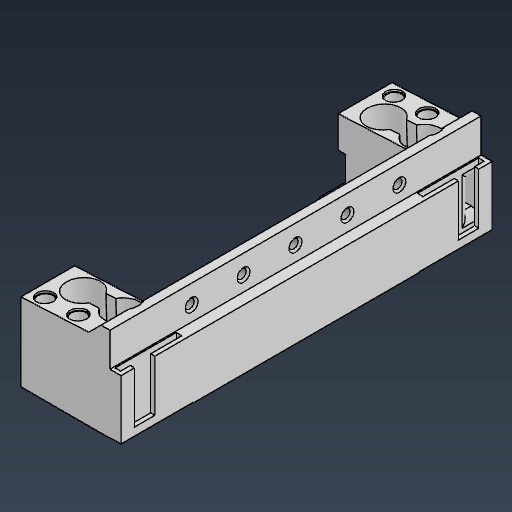
# Autodesk Inventor part: FonrtMount
Saved by Autodesk Inventor 2026.2 (Build 302298010, 298A)
## iProperties
Created: 2026-04-04
Part Number: FonrtMount
Material: Generic
Document SubType Name: Modeling
Designer: szymo
Density: 1 g/cm^3
Appearance: Default
Author: szymo
Autodesk Inventor part; units mm, degrees
(part 1 of 2)
ref_plane "YZ Plane" through (0, 0, 0) normal (1, 0, 0) x (0, 1, 0)
ref_plane "XZ Plane" through (0, 0, 0) normal (0, 1, 0) x (-1, 0, 0)
ref_plane "XY Plane" through (0, 0, 0) normal (0, 0, 1) x (1, 0, 0)
sketch "Sketch1" plane through (0, 0, 0) normal (0, 0, 1) x (1, 0, 0)
  line L0 (-27, 86.2958) -> (-6.5, 86.2958) projected
  line L1 (-6.5, 86.2958) -> (-6.5, 69.7958) projected
  line L2 (-27, 69.7958) -> (-6.5, 69.7958) projected
  line L3 (-27, 86.2958) -> (-27, 69.7958) projected
  line L4 (0, 95.9) -> (0, 81.9) projected
  line L5 (0, 81.9) -> (-3, 81.9) projected
  line L6 (-3, 81.9) -> (-3, 90.9) projected
  line L7 (-3, 90.9) -> (-5, 90.9) projected
  line L8 (-5, 90.9) -> (0, 95.9) projected
  circle A0 centre (-14.5, 55.2958) radius 14.5 projected
  line L9 (-9.2042, 86.6958) -> (-6, 86.6958)
  line L10 (-6, 86.6958) -> (-6, 69.2958)
  line L11 (-6, 69.2958) -> (-10.7251, 69.2958)
  line L12 (-4, 65.2958) -> (0, 65.2958)
  line L13 (0, 65.2958) -> (0, 81.4)
  line L14 (0, 81.4) -> (-3, 81.4)
  line L15 (-3, 81.4) -> (-3, 90.5)
  line L16 (-5.4, 90.5) -> (-9.2042, 86.6958)
  line L17 (-5.4, 90.5) -> (-3, 90.5)
  line L18 (-5.4, 90.5) -> (-5, 90.9) construction
  line L19 (-9.2085, 69.2958) -> (-9.2085, 68.7958)
  line L20 (-8.7042, 87.1958) -> (-8.7042, 86.6958)
  arc A1 (-5.2144, 40.6176) -> (-6.571, 40.1714) centre (-4.0302, 34.7325) ccw construction
  arc A2 (-4.9311, 40.2025) -> (-5.2144, 40.6176) centre (-13, 35.0012) ccw construction
  arc A3 (-5.8414, 39.102) -> (-4.9311, 40.2025) centre (-9.9791, 43.4512) ccw construction
  arc A4 (-5.6366, 38.7217) -> (-5.8414, 39.102) centre (-13, 35.0012) ccw construction
  arc A5 (-4.2168, 38.8762) -> (-5.6366, 38.7217) centre (-4.2821, 32.8735) ccw construction
  arc A6 (-4.026, 38.4112) -> (-4.2168, 38.8762) centre (-13, 35.0012) ccw construction
  arc A7 (-5.1452, 37.524) -> (-4.026, 38.4112) centre (-8.2882, 42.6385) ccw construction
  arc A8 (-5.0239, 37.1095) -> (-5.1452, 37.524) centre (-13, 35.0012) ccw construction
  arc A9 (-3.6031, 36.9654) -> (-5.0239, 37.1095) centre (-4.915, 31.1074) ccw construction
  arc A10 (-3.5132, 36.4709) -> (-3.6031, 36.9654) centre (-13, 35.0012) ccw construction
  arc A11 (-4.7923, 35.8358) -> (-3.5132, 36.4709) centre (-6.8033, 41.492) ccw construction
  arc A12 (-4.7599, 35.4051) -> (-4.7923, 35.8358) centre (-13, 35.0012) ccw construction
  arc A13 (-3.4001, 34.9687) -> (-4.7599, 35.4051) centre (-5.9012, 29.5115) ccw construction
  arc A14 (-3.4149, 34.4663) -> (-3.4001, 34.9687) centre (-13, 35.0012) ccw construction
  arc A15 (-4.7982, 34.1111) -> (-3.4149, 34.4663) centre (-5.5892, 40.0618) ccw construction
  arc A16 (-4.856, 33.6831) -> (-4.7982, 34.1111) centre (-13, 35.0012) ccw construction
  arc A17 (-3.6166, 32.9735) -> (-4.856, 33.6831) centre (-7.1977, 28.1556) ccw construction
  arc A18 (-3.7356, 32.4852) -> (-3.6166, 32.9735) centre (-13, 35.0012) ccw construction
  arc A19 (-5.1625, 32.4253) -> (-3.7356, 32.4852) centre (-4.699, 38.4104) ccw construction
  arc A20 (-5.308, 32.0186) -> (-5.1625, 32.4253) centre (-13, 35.0012) ccw construction
  arc A21 (-4.2432, 31.0669) -> (-5.308, 32.0186) centre (-8.7478, 27.0988) ccw construction
  arc A22 (-4.4611, 30.614) -> (-4.2432, 31.0669) centre (-13, 35.0012) ccw construction
  arc A23 (-5.8693, 30.8521) -> (-4.4611, 30.614) centre (-4.1716, 36.61) ccw construction
  arc A24 (-6.0962, 30.4845) -> (-5.8693, 30.8521) centre (-13, 35.0012) ccw construction
  arc A25 (-5.2526, 29.3322) -> (-6.0962, 30.4845) centre (-10.4837, 26.3874) ccw construction
  arc A26 (-5.5599, 28.9345) -> (-5.2526, 29.3322) centre (-13, 35.0012) ccw construction
  arc A27 (-6.8878, 29.4602) -> (-5.5599, 28.9345) centre (-4.03, 34.7394) ccw construction
  arc A28 (-7.1861, 29.1479) -> (-6.8878, 29.4602) centre (-13, 35.0012) ccw construction
  arc A29 (-6.6005, 27.8453) -> (-7.1861, 29.1479) centre (-12.3296, 26.0525) ccw construction
  arc A30 (-6.9838, 27.5202) -> (-6.6005, 27.8453) centre (-13, 35.0012) ccw construction
  arc A31 (-8.1734, 28.3104) -> (-6.9838, 27.5202) centre (-4.2805, 32.8801) ccw construction
  arc A32 (-8.5302, 28.067) -> (-8.1734, 28.3104) centre (-13, 35.0012) ccw construction
  arc A33 (-8.2282, 26.6712) -> (-8.5302, 28.067) centre (-14.2048, 26.1086) ccw construction
  arc A34 (-8.6707, 26.4328) -> (-8.2282, 26.6712) centre (-13, 35.0012) ccw construction
  arc A35 (-9.6699, 27.4531) -> (-8.6707, 26.4328) centre (-4.912, 31.1136) ccw construction
  arc A36 (-10.0695, 27.2892) -> (-9.6699, 27.4531) centre (-13, 35.0012) ccw construction
  arc A37 (-10.0643, 25.8611) -> (-10.0695, 27.2892) centre (-16.0273, 26.5534) ccw construction
  arc A38 (-10.5467, 25.72) -> (-10.0643, 25.8611) centre (-13, 35.0012) ccw construction
  arc A39 (-11.312, 26.9257) -> (-10.5467, 25.72) centre (-5.897, 29.5169) ccw construction
  arc A40 (-11.737, 26.8485) -> (-11.312, 26.9257) centre (-13, 35.0012) ccw construction
  arc A41 (-12.0288, 25.4504) -> (-11.737, 26.8485) centre (-17.7176, 27.3675) ccw construction
  arc A42 (-12.53, 25.4127) -> (-12.0288, 25.4504) centre (-13, 35.0012) ccw construction
  arc A43 (-13.0279, 26.7512) -> (-12.53, 25.4127) centre (-7.1925, 28.16) ccw construction
  arc A44 (-13.4596, 26.764) -> (-13.0279, 26.7512) centre (-13, 35.0012) ccw construction
  arc A45 (-14.0358, 25.4572) -> (-13.4596, 26.764) centre (-19.2016, 28.5151) ccw construction
  arc A46 (-14.5338, 25.5245) -> (-14.0358, 25.4572) centre (-13, 35.0012) ccw construction
  arc A47 (-14.7426, 26.9373) -> (-14.5338, 25.5245) centre (-8.7418, 27.102) ccw construction
  arc A48 (-15.1622, 27.0396) -> (-14.7426, 26.9373) centre (-13, 35.0012) ccw construction
  arc A49 (-15.9974, 25.8811) -> (-15.1622, 27.0396) centre (-20.4146, 29.9462) ccw construction
  arc A50 (-16.4706, 26.0505) -> (-15.9974, 25.8811) centre (-13, 35.0012) ccw construction
  arc A51 (-16.3811, 27.4758) -> (-16.4706, 26.0505) centre (-10.4772, 26.3893) ccw construction
  arc A52 (-16.7703, 27.6631) -> (-16.3811, 27.4758) centre (-13, 35.0012) ccw construction
  arc A53 (-17.8281, 26.7036) -> (-16.7703, 27.6631) centre (-21.3036, 31.5983) ccw construction
  arc A54 (-18.2557, 26.9677) -> (-17.8281, 26.7036) centre (-13, 35.0012) ccw construction
  arc A55 (-17.8718, 28.3432) -> (-18.2557, 26.9677) centre (-12.3228, 26.053) ccw construction
  arc A56 (-18.2136, 28.6073) -> (-17.8718, 28.3432) centre (-13, 35.0012) ccw construction
  arc A57 (-19.4477, 27.8888) -> (-18.2136, 28.6073) centre (-21.8296, 33.3991) ccw construction
  arc A58 (-19.8111, 28.236) -> (-19.4477, 27.8888) centre (-13, 35.0012) ccw construction
  arc A59 (-19.1496, 29.5016) -> (-19.8111, 28.236) centre (-14.198, 26.1077) ccw construction
  arc A60 (-19.429, 29.831) -> (-19.1496, 29.5016) centre (-13, 35.0012) ccw construction
  arc A61 (-20.7856, 29.3848) -> (-19.429, 29.831) centre (-21.9698, 35.2699) ccw construction
  arc A62 (-21.0689, 29.7999) -> (-20.7856, 29.3848) centre (-13, 35.0012) ccw construction
  arc A63 (-20.1586, 30.9004) -> (-21.0689, 29.7999) centre (-16.0209, 26.5512) ccw construction
  arc A64 (-20.3634, 31.2807) -> (-20.1586, 30.9004) centre (-13, 35.0012) ccw construction
  arc A65 (-21.7832, 31.1262) -> (-20.3634, 31.2807) centre (-21.7179, 37.1289) ccw construction
  arc A66 (-21.974, 31.5912) -> (-21.7832, 31.1262) centre (-13, 35.0012) ccw construction
  arc A67 (-20.8548, 32.4784) -> (-21.974, 31.5912) centre (-17.7118, 27.3639) ccw construction
  arc A68 (-20.9761, 32.8929) -> (-20.8548, 32.4784) centre (-13, 35.0012) ccw construction
  arc A69 (-22.3969, 33.037) -> (-20.9761, 32.8929) centre (-21.085, 38.895) ccw construction
  arc A70 (-22.4868, 33.5315) -> (-22.3969, 33.037) centre (-13, 35.0012) ccw construction
  arc A71 (-21.2077, 34.1666) -> (-22.4868, 33.5315) centre (-19.1967, 28.5104) ccw construction
  arc A72 (-21.2401, 34.5973) -> (-21.2077, 34.1666) centre (-13, 35.0012) ccw construction
  arc A73 (-22.5999, 35.0337) -> (-21.2401, 34.5973) centre (-20.0988, 40.4909) ccw construction
  arc A74 (-22.5851, 35.5361) -> (-22.5999, 35.0337) centre (-13, 35.0012) ccw construction
  arc A75 (-21.2018, 35.8913) -> (-22.5851, 35.5361) centre (-20.4108, 29.9406) ccw construction
  arc A76 (-21.144, 36.3193) -> (-21.2018, 35.8913) centre (-13, 35.0012) ccw construction
  arc A77 (-22.3834, 37.0289) -> (-21.144, 36.3193) centre (-18.8023, 41.8468) ccw construction
  arc A78 (-22.2644, 37.5172) -> (-22.3834, 37.0289) centre (-13, 35.0012) ccw construction
  arc A79 (-20.8375, 37.5771) -> (-22.2644, 37.5172) centre (-21.301, 31.592) ccw construction
  arc A80 (-20.692, 37.9838) -> (-20.8375, 37.5771) centre (-13, 35.0012) ccw construction
  arc A81 (-21.7568, 38.9355) -> (-20.692, 37.9838) centre (-17.2522, 42.9036) ccw construction
  arc A82 (-21.5389, 39.3884) -> (-21.7568, 38.9355) centre (-13, 35.0012) ccw construction
  arc A83 (-20.1307, 39.1503) -> (-21.5389, 39.3884) centre (-21.8284, 33.3924) ccw construction
  arc A84 (-19.9038, 39.5178) -> (-20.1307, 39.1503) centre (-13, 35.0012) ccw construction
  arc A85 (-20.7474, 40.6702) -> (-19.9038, 39.5178) centre (-15.5163, 43.615) ccw construction
  arc A86 (-20.4401, 41.0679) -> (-20.7474, 40.6702) centre (-13, 35.0012) ccw construction
  arc A87 (-19.1122, 40.5422) -> (-20.4401, 41.0679) centre (-21.97, 35.263) ccw construction
  arc A88 (-18.8139, 40.8545) -> (-19.1122, 40.5422) centre (-13, 35.0012) ccw construction
  arc A89 (-19.3995, 42.1571) -> (-18.8139, 40.8545) centre (-13.6704, 43.9499) ccw construction
  arc A90 (-19.0162, 42.4822) -> (-19.3995, 42.1571) centre (-13, 35.0012) ccw construction
  arc A91 (-17.8266, 41.692) -> (-19.0162, 42.4822) centre (-21.7195, 37.1223) ccw construction
  arc A92 (-17.4698, 41.9354) -> (-17.8266, 41.692) centre (-13, 35.0012) ccw construction
  arc A93 (-17.7718, 43.3312) -> (-17.4698, 41.9354) centre (-11.7952, 43.8938) ccw construction
  arc A94 (-17.3293, 43.5696) -> (-17.7718, 43.3312) centre (-13, 35.0012) ccw construction
  arc A95 (-16.3301, 42.5493) -> (-17.3293, 43.5696) centre (-21.088, 38.8888) ccw construction
  arc A96 (-15.9305, 42.7132) -> (-16.3301, 42.5493) centre (-13, 35.0012) ccw construction
  arc A97 (-15.9357, 44.1413) -> (-15.9305, 42.7132) centre (-9.9727, 43.4489) ccw construction
  arc A98 (-15.4533, 44.2824) -> (-15.9357, 44.1413) centre (-13, 35.0012) ccw construction
  arc A99 (-14.688, 43.0767) -> (-15.4533, 44.2824) centre (-20.103, 40.4855) ccw construction
  arc A100 (-14.263, 43.1539) -> (-14.688, 43.0767) centre (-13, 35.0012) ccw construction
  arc A101 (-13.9712, 44.5519) -> (-14.263, 43.1539) centre (-8.2824, 42.6349) ccw construction
  arc A102 (-13.47, 44.5897) -> (-13.9712, 44.5519) centre (-13, 35.0012) ccw construction
  arc A103 (-12.9721, 43.2512) -> (-13.47, 44.5897) centre (-18.8075, 41.8424) ccw construction
  arc A104 (-12.5404, 43.2384) -> (-12.9721, 43.2512) centre (-13, 35.0012) ccw construction
  arc A105 (-11.9642, 44.5452) -> (-12.5404, 43.2384) centre (-6.7984, 41.4873) ccw construction
  arc A106 (-11.4662, 44.4779) -> (-11.9642, 44.5452) centre (-13, 35.0012) ccw construction
  arc A107 (-11.2574, 43.0651) -> (-11.4662, 44.4779) centre (-17.2582, 42.9004) ccw construction
  arc A108 (-10.8378, 42.9628) -> (-11.2574, 43.0651) centre (-13, 35.0012) ccw construction
  arc A109 (-10.0026, 44.1213) -> (-10.8378, 42.9628) centre (-5.5854, 40.0562) ccw construction
  arc A110 (-9.5294, 43.9519) -> (-10.0026, 44.1213) centre (-13, 35.0012) ccw construction
  arc A111 (-9.6189, 42.5266) -> (-9.5294, 43.9519) centre (-15.5228, 43.6131) ccw construction
  arc A112 (-9.2297, 42.3393) -> (-9.6189, 42.5266) centre (-13, 35.0012) ccw construction
  arc A113 (-8.1719, 43.2988) -> (-9.2297, 42.3393) centre (-4.6964, 38.4041) ccw construction
  arc A114 (-7.7443, 43.0347) -> (-8.1719, 43.2988) centre (-13, 35.0012) ccw construction
  arc A115 (-8.1282, 41.6591) -> (-7.7443, 43.0347) centre (-13.6772, 43.9494) ccw construction
  arc A116 (-7.7864, 41.3951) -> (-8.1282, 41.6591) centre (-13, 35.0012) ccw construction
  arc A117 (-6.5523, 42.1136) -> (-7.7864, 41.3951) centre (-4.1704, 36.6033) ccw construction
  arc A118 (-6.1889, 41.7664) -> (-6.5523, 42.1136) centre (-13, 35.0012) ccw construction
  arc A119 (-6.8504, 40.5008) -> (-6.1889, 41.7664) centre (-11.802, 43.8947) ccw construction
  arc A120 (-6.571, 40.1714) -> (-6.8504, 40.5008) centre (-13, 35.0012) ccw construction
  circle A121 centre (-13, 35.0012) radius 9.6 construction
  line L21 (-4, 65.2958) -> (-27, 65.2958)
  line L22 (-27, 65.2958) -> (-27, 24.2538) construction
  line L23 (-27, 65.2958) -> (-27, 69.2958)
  line L24 (-27, 69.2958) -> (-9.2085, 69.2958)
  point P0 (0, 0)
  dimension "d0" = 4.5
  dimension "d1" = 0.5
  dimension "d2" = 0.5
  dimension "d3" = 0.4
  dimension "d4" = 45
  dimension "d5" = 0.4
  dimension "d6" = 0.5
  dimension "d11" = 0.5
  dimension "d12" = 0.5
  dimension "d32" = 2
  constraints: 32 end point, 7 perpendicular, 4 point on line, 3 horizontal, 3 point on circle, 3 vertical, 2 collinear, 1 coincident, 1 tangent, 3 other
  measures "d0" distance between parallel lines of L12 L2
  measures "d1" distance between parallel lines of L2 L11
  measures "d2" distance between parallel lines of L1 L10
  measures "d3" distance between parallel lines of L9 L0
  measures "d4" angle of L9 L16
  measures "d5" distance between parallel lines of L7 L17
  measures "d6" distance between parallel lines of L5 L14
  measures "d11" distance of L19.start L19.end
  measures "d12" distance of L20.start L20.end
  measures "d32" distance edge to line of A0 L22
extrude "Extrusion2" add sketch "Sketch1" along normal blind 19 and the other way blind 18.4 contours L19 L11 L10 L9 L20 L16 L17 L6 L15 L14 L13 L12 A0
sketch "Sketch2" plane through (0, 0, -18.4) normal (0, 0, -1) x (-1, 0, 0)
  arc A0 (6.571, 40.1714) -> (5.2144, 40.6176) centre (4.0302, 34.7325) ccw construction
  arc A1 (5.2144, 40.6176) -> (4.9311, 40.2025) centre (13, 35.0012) ccw construction
  arc A2 (4.9311, 40.2025) -> (5.8414, 39.102) centre (9.9791, 43.4512) ccw construction
  arc A3 (5.8414, 39.102) -> (5.6366, 38.7217) centre (13, 35.0012) ccw construction
  arc A4 (5.6366, 38.7217) -> (4.2168, 38.8762) centre (4.2821, 32.8735) ccw construction
  arc A5 (4.2168, 38.8762) -> (4.026, 38.4112) centre (13, 35.0012) ccw construction
  arc A6 (4.026, 38.4112) -> (5.1452, 37.524) centre (8.2882, 42.6385) ccw construction
  arc A7 (5.1452, 37.524) -> (5.0239, 37.1095) centre (13, 35.0012) ccw construction
  arc A8 (5.0239, 37.1095) -> (3.6031, 36.9654) centre (4.915, 31.1074) ccw construction
  arc A9 (3.6031, 36.9654) -> (3.5132, 36.4709) centre (13, 35.0012) ccw construction
  arc A10 (3.5132, 36.4709) -> (4.7923, 35.8358) centre (6.8033, 41.492) ccw construction
  arc A11 (4.7923, 35.8358) -> (4.7599, 35.4051) centre (13, 35.0012) ccw construction
  arc A12 (4.7599, 35.4051) -> (3.4001, 34.9687) centre (5.9012, 29.5115) ccw construction
  arc A13 (3.4001, 34.9687) -> (3.4149, 34.4663) centre (13, 35.0012) ccw construction
  arc A14 (3.4149, 34.4663) -> (4.7982, 34.1111) centre (5.5892, 40.0618) ccw construction
  arc A15 (4.7982, 34.1111) -> (4.856, 33.6831) centre (13, 35.0012) ccw construction
  arc A16 (4.856, 33.6831) -> (3.6166, 32.9735) centre (7.1977, 28.1556) ccw construction
  arc A17 (3.6166, 32.9735) -> (3.7356, 32.4852) centre (13, 35.0012) ccw construction
  arc A18 (3.7356, 32.4852) -> (5.1625, 32.4253) centre (4.699, 38.4104) ccw construction
  arc A19 (5.1625, 32.4253) -> (5.308, 32.0186) centre (13, 35.0012) ccw construction
  arc A20 (5.308, 32.0186) -> (4.2432, 31.0669) centre (8.7478, 27.0988) ccw construction
  arc A21 (4.2432, 31.0669) -> (4.4611, 30.614) centre (13, 35.0012) ccw construction
  arc A22 (4.4611, 30.614) -> (5.8693, 30.8521) centre (4.1716, 36.61) ccw construction
  arc A23 (5.8693, 30.8521) -> (6.0962, 30.4845) centre (13, 35.0012) ccw construction
  arc A24 (6.0962, 30.4845) -> (5.2526, 29.3322) centre (10.4837, 26.3874) ccw construction
  arc A25 (5.2526, 29.3322) -> (5.5599, 28.9345) centre (13, 35.0012) ccw construction
  arc A26 (5.5599, 28.9345) -> (6.8878, 29.4602) centre (4.03, 34.7394) ccw construction
  arc A27 (6.8878, 29.4602) -> (7.1861, 29.1479) centre (13, 35.0012) ccw construction
  arc A28 (7.1861, 29.1479) -> (6.6005, 27.8453) centre (12.3296, 26.0525) ccw construction
  arc A29 (6.6005, 27.8453) -> (6.9838, 27.5202) centre (13, 35.0012) ccw construction
  arc A30 (6.9838, 27.5202) -> (8.1734, 28.3104) centre (4.2805, 32.8801) ccw construction
  arc A31 (8.1734, 28.3104) -> (8.5302, 28.067) centre (13, 35.0012) ccw construction
  arc A32 (8.5302, 28.067) -> (8.2282, 26.6712) centre (14.2048, 26.1086) ccw construction
  arc A33 (8.2282, 26.6712) -> (8.6707, 26.4328) centre (13, 35.0012) ccw construction
  arc A34 (8.6707, 26.4328) -> (9.6699, 27.4531) centre (4.912, 31.1136) ccw construction
  arc A35 (9.6699, 27.4531) -> (10.0695, 27.2892) centre (13, 35.0012) ccw construction
  arc A36 (10.0695, 27.2892) -> (10.0643, 25.8611) centre (16.0273, 26.5534) ccw construction
  arc A37 (10.0643, 25.8611) -> (10.5467, 25.72) centre (13, 35.0012) ccw construction
  arc A38 (10.5467, 25.72) -> (11.312, 26.9257) centre (5.897, 29.5169) ccw construction
  arc A39 (11.312, 26.9257) -> (11.737, 26.8485) centre (13, 35.0012) ccw construction
  arc A40 (11.737, 26.8485) -> (12.0288, 25.4504) centre (17.7176, 27.3675) ccw construction
  arc A41 (12.0288, 25.4504) -> (12.53, 25.4127) centre (13, 35.0012) ccw construction
  arc A42 (12.53, 25.4127) -> (13.0279, 26.7512) centre (7.1925, 28.16) ccw construction
  arc A43 (13.0279, 26.7512) -> (13.4596, 26.764) centre (13, 35.0012) ccw construction
  arc A44 (13.4596, 26.764) -> (14.0358, 25.4572) centre (19.2016, 28.5151) ccw construction
  arc A45 (14.0358, 25.4572) -> (14.5338, 25.5245) centre (13, 35.0012) ccw construction
  arc A46 (14.5338, 25.5245) -> (14.7426, 26.9373) centre (8.7418, 27.102) ccw construction
  arc A47 (14.7426, 26.9373) -> (15.1622, 27.0396) centre (13, 35.0012) ccw construction
  arc A48 (15.1622, 27.0396) -> (15.9974, 25.8811) centre (20.4146, 29.9462) ccw construction
  arc A49 (15.9974, 25.8811) -> (16.4706, 26.0505) centre (13, 35.0012) ccw construction
  arc A50 (16.4706, 26.0505) -> (16.3811, 27.4758) centre (10.4772, 26.3893) ccw construction
  arc A51 (16.3811, 27.4758) -> (16.7703, 27.6631) centre (13, 35.0012) ccw construction
  arc A52 (16.7703, 27.6631) -> (17.8281, 26.7036) centre (21.3036, 31.5983) ccw construction
  arc A53 (17.8281, 26.7036) -> (18.2557, 26.9677) centre (13, 35.0012) ccw construction
  arc A54 (18.2557, 26.9677) -> (17.8718, 28.3432) centre (12.3228, 26.053) ccw construction
  arc A55 (17.8718, 28.3432) -> (18.2136, 28.6073) centre (13, 35.0012) ccw construction
  arc A56 (18.2136, 28.6073) -> (19.4477, 27.8888) centre (21.8296, 33.3991) ccw construction
  arc A57 (19.4477, 27.8888) -> (19.8111, 28.236) centre (13, 35.0012) ccw construction
  arc A58 (19.8111, 28.236) -> (19.1496, 29.5016) centre (14.198, 26.1077) ccw construction
  arc A59 (19.1496, 29.5016) -> (19.429, 29.831) centre (13, 35.0012) ccw construction
  arc A60 (19.429, 29.831) -> (20.7856, 29.3848) centre (21.9698, 35.2699) ccw construction
  arc A61 (20.7856, 29.3848) -> (21.0689, 29.7999) centre (13, 35.0012) ccw construction
  arc A62 (21.0689, 29.7999) -> (20.1586, 30.9004) centre (16.0209, 26.5512) ccw construction
  arc A63 (20.1586, 30.9004) -> (20.3634, 31.2807) centre (13, 35.0012) ccw construction
  arc A64 (20.3634, 31.2807) -> (21.7832, 31.1262) centre (21.7179, 37.1289) ccw construction
  arc A65 (21.7832, 31.1262) -> (21.974, 31.5912) centre (13, 35.0012) ccw construction
  arc A66 (21.974, 31.5912) -> (20.8548, 32.4784) centre (17.7118, 27.3639) ccw construction
  arc A67 (20.8548, 32.4784) -> (20.9761, 32.8929) centre (13, 35.0012) ccw construction
  arc A68 (20.9761, 32.8929) -> (22.3969, 33.037) centre (21.085, 38.895) ccw construction
  arc A69 (22.3969, 33.037) -> (22.4868, 33.5315) centre (13, 35.0012) ccw construction
  arc A70 (22.4868, 33.5315) -> (21.2077, 34.1666) centre (19.1967, 28.5104) ccw construction
  arc A71 (21.2077, 34.1666) -> (21.2401, 34.5973) centre (13, 35.0012) ccw construction
  arc A72 (21.2401, 34.5973) -> (22.5999, 35.0337) centre (20.0988, 40.4909) ccw construction
  arc A73 (22.5999, 35.0337) -> (22.5851, 35.5361) centre (13, 35.0012) ccw construction
  arc A74 (22.5851, 35.5361) -> (21.2018, 35.8913) centre (20.4108, 29.9406) ccw construction
  arc A75 (21.2018, 35.8913) -> (21.144, 36.3193) centre (13, 35.0012) ccw construction
  arc A76 (21.144, 36.3193) -> (22.3834, 37.0289) centre (18.8023, 41.8468) ccw construction
  arc A77 (22.3834, 37.0289) -> (22.2644, 37.5172) centre (13, 35.0012) ccw construction
  arc A78 (22.2644, 37.5172) -> (20.8375, 37.5771) centre (21.301, 31.592) ccw construction
  arc A79 (20.8375, 37.5771) -> (20.692, 37.9838) centre (13, 35.0012) ccw construction
  arc A80 (20.692, 37.9838) -> (21.7568, 38.9355) centre (17.2522, 42.9036) ccw construction
  arc A81 (21.7568, 38.9355) -> (21.5389, 39.3884) centre (13, 35.0012) ccw construction
  arc A82 (21.5389, 39.3884) -> (20.1307, 39.1503) centre (21.8284, 33.3924) ccw construction
  arc A83 (20.1307, 39.1503) -> (19.9038, 39.5178) centre (13, 35.0012) ccw construction
  arc A84 (19.9038, 39.5178) -> (20.7474, 40.6702) centre (15.5163, 43.615) ccw construction
  arc A85 (20.7474, 40.6702) -> (20.4401, 41.0679) centre (13, 35.0012) ccw construction
  arc A86 (20.4401, 41.0679) -> (19.1122, 40.5422) centre (21.97, 35.263) ccw construction
  arc A87 (19.1122, 40.5422) -> (18.8139, 40.8545) centre (13, 35.0012) ccw construction
  arc A88 (18.8139, 40.8545) -> (19.3995, 42.1571) centre (13.6704, 43.9499) ccw construction
  arc A89 (19.3995, 42.1571) -> (19.0162, 42.4822) centre (13, 35.0012) ccw construction
  arc A90 (19.0162, 42.4822) -> (17.8266, 41.692) centre (21.7195, 37.1223) ccw construction
  arc A91 (17.8266, 41.692) -> (17.4698, 41.9354) centre (13, 35.0012) ccw construction
  arc A92 (17.4698, 41.9354) -> (17.7718, 43.3312) centre (11.7952, 43.8938) ccw construction
  arc A93 (17.7718, 43.3312) -> (17.3293, 43.5696) centre (13, 35.0012) ccw construction
  arc A94 (17.3293, 43.5696) -> (16.3301, 42.5493) centre (21.088, 38.8888) ccw construction
  arc A95 (16.3301, 42.5493) -> (15.9305, 42.7132) centre (13, 35.0012) ccw construction
  arc A96 (15.9305, 42.7132) -> (15.9357, 44.1413) centre (9.9727, 43.4489) ccw construction
  arc A97 (15.9357, 44.1413) -> (15.4533, 44.2824) centre (13, 35.0012) ccw construction
  arc A98 (15.4533, 44.2824) -> (14.688, 43.0767) centre (20.103, 40.4855) ccw construction
  arc A99 (14.688, 43.0767) -> (14.263, 43.1539) centre (13, 35.0012) ccw construction
  arc A100 (14.263, 43.1539) -> (13.9712, 44.5519) centre (8.2824, 42.6349) ccw construction
  arc A101 (13.9712, 44.5519) -> (13.47, 44.5897) centre (13, 35.0012) ccw construction
  arc A102 (13.47, 44.5897) -> (12.9721, 43.2512) centre (18.8075, 41.8424) ccw construction
  arc A103 (12.9721, 43.2512) -> (12.5404, 43.2384) centre (13, 35.0012) ccw construction
  arc A104 (12.5404, 43.2384) -> (11.9642, 44.5452) centre (6.7984, 41.4873) ccw construction
  arc A105 (11.9642, 44.5452) -> (11.4662, 44.4779) centre (13, 35.0012) ccw construction
  arc A106 (11.4662, 44.4779) -> (11.2574, 43.0651) centre (17.2582, 42.9004) ccw construction
  arc A107 (11.2574, 43.0651) -> (10.8378, 42.9628) centre (13, 35.0012) ccw construction
  arc A108 (10.8378, 42.9628) -> (10.0026, 44.1213) centre (5.5854, 40.0562) ccw construction
  arc A109 (10.0026, 44.1213) -> (9.5294, 43.9519) centre (13, 35.0012) ccw construction
  arc A110 (9.5294, 43.9519) -> (9.6189, 42.5266) centre (15.5228, 43.6131) ccw construction
  arc A111 (9.6189, 42.5266) -> (9.2297, 42.3393) centre (13, 35.0012) ccw construction
  arc A112 (9.2297, 42.3393) -> (8.1719, 43.2988) centre (4.6964, 38.4041) ccw construction
  arc A113 (8.1719, 43.2988) -> (7.7443, 43.0347) centre (13, 35.0012) ccw construction
  arc A114 (7.7443, 43.0347) -> (8.1282, 41.6591) centre (13.6772, 43.9494) ccw construction
  arc A115 (8.1282, 41.6591) -> (7.7864, 41.3951) centre (13, 35.0012) ccw construction
  arc A116 (7.7864, 41.3951) -> (6.5523, 42.1136) centre (4.1704, 36.6033) ccw construction
  arc A117 (6.5523, 42.1136) -> (6.1889, 41.7664) centre (13, 35.0012) ccw construction
  arc A118 (6.1889, 41.7664) -> (6.8504, 40.5008) centre (11.802, 43.8947) ccw construction
  arc A119 (6.8504, 40.5008) -> (6.571, 40.1714) centre (13, 35.0012) ccw construction
  circle A120 centre (13, 35.0012) radius 9.6 construction
  line L0 (23.8, 32.6031) -> (23.8, 65.2958) construction
  line L1 (9.2085, 69.2958) -> (6, 69.2958) projected
  line L2 (6, 69.2958) -> (6, 86.6958) projected
  line L3 (6, 86.6958) -> (8.7042, 86.6958) projected
  line L4 (8.7042, 86.6958) -> (8.7042, 87.1958) projected
  line L5 (8.7042, 87.1958) -> (5.4, 90.5) projected
  line L6 (5.4, 90.5) -> (3, 90.5) projected
  line L7 (3, 90.5) -> (3, 81.4) projected
  line L8 (3, 81.4) -> (0, 81.4) projected
  line L9 (0, 81.4) -> (0, 65.2958) projected
  line L10 (0, 65.2958) -> (4, 65.2958) projected
  arc A121 (9.2085, 68.7958) -> (4, 65.2958) centre (14.5, 55.2958) ccw projected
  line L11 (9.2085, 68.7958) -> (9.2085, 69.2958) projected
  line L12 (4, 65.2958) -> (23.8, 65.2958)
  line L13 (23.8, 65.2958) -> (23.8, 69.2958)
  line L14 (23.8, 69.2958) -> (9.2085, 69.2958)
  circle A122 centre (14.5, 55.2958) radius 14.5 projected
  point P0 (0, 0)
  dimension "d33" = 5.2
  dimension "d35" = 1.2
  constraints: 8 end point, 2 vertical, 1 coincident, 1 horizontal, 1 perpendicular, 3 other
  measures "d33" distance edge to line of A122 L0
extrude "Extrusion3" add sketch "Sketch2" along normal blind 17.1 contours L11 A121 L10 L9 L8 L7 L6 L5 L4 L3 L2 L1 | L14 A122 L11 | A122 L14 L13 L12 A121 | L14 L13 A122
sketch "Sketch3" plane through (0, 0, 19) normal (0, 0, 1) x (1, 0, 0)
  arc A0 (-20.6322, 38.1335) -> (-22.0597, 38.1763) centre (-21.5245, 32.1971) ccw construction
  arc A1 (-22.0597, 38.1763) -> (-22.2135, 37.6978) centre (-13, 35.0012) ccw construction
  arc A2 (-22.2135, 37.6978) -> (-21.0283, 36.901) centre (-18.2955, 42.246) ccw construction
  arc A3 (-21.0283, 36.901) -> (-21.1167, 36.4782) centre (-13, 35.0012) ccw construction
  arc A4 (-21.1167, 36.4782) -> (-22.5219, 36.2233) centre (-20.7552, 30.4861) ccw construction
  arc A5 (-22.5219, 36.2233) -> (-22.5728, 35.7233) centre (-13, 35.0012) ccw construction
  arc A6 (-22.5728, 35.7233) -> (-21.2478, 35.1903) centre (-19.6861, 40.9866) ccw construction
  arc A7 (-21.2478, 35.1903) -> (-21.2464, 34.7584) centre (-13, 35.0012) ccw construction
  arc A8 (-21.2464, 34.7584) -> (-22.5679, 34.2168) centre (-19.647, 28.9724) ccw construction
  arc A9 (-22.5679, 34.2168) -> (-22.5137, 33.7172) centre (-13, 35.0012) ccw construction
  arc A10 (-22.5137, 33.7172) -> (-21.1069, 33.4714) centre (-20.7844, 39.4657) ccw construction
  arc A11 (-21.1069, 33.4714) -> (-21.0157, 33.0492) centre (-13, 35.0012) ccw construction
  arc A12 (-21.0157, 33.0492) -> (-22.1957, 32.2447) centre (-18.2483, 27.7221) ccw construction
  arc A13 (-22.1957, 32.2447) -> (-22.0389, 31.7672) centre (-13, 35.0012) ccw construction
  arc A14 (-22.0389, 31.7672) -> (-20.6117, 31.8193) centre (-21.5425, 37.7497) ccw construction
  arc A15 (-20.6117, 31.8193) -> (-20.4347, 31.4253) centre (-13, 35.0012) ccw construction
  arc A16 (-20.4347, 31.4253) -> (-21.4217, 30.393) centre (-16.6202, 26.79) ccw construction
  arc A17 (-21.4217, 30.393) -> (-21.169, 29.9586) centre (-13, 35.0012) ccw construction
  arc A18 (-21.169, 29.9586) -> (-19.7838, 30.3062) centre (-21.9273, 35.9136) ccw construction
  arc A19 (-19.7838, 30.3062) -> (-19.5288, 29.9576) centre (-13, 35.0012) ccw construction
  arc A20 (-19.5288, 29.9576) -> (-20.2796, 28.7428) centre (-14.8338, 26.2168) ccw construction
  arc A21 (-20.2796, 28.7428) -> (-19.9421, 28.3704) centre (-13, 35.0012) ccw construction
  arc A22 (-19.9421, 28.3704) -> (-18.6594, 28.9984) centre (-21.9219, 34.0375) ccw construction
  arc A23 (-18.6594, 28.9984) -> (-18.3375, 28.7104) centre (-13, 35.0012) ccw construction
  arc A24 (-18.3375, 28.7104) -> (-18.8193, 27.366) centre (-12.9674, 26.0275) ccw construction
  arc A25 (-18.8193, 27.366) -> (-18.4117, 27.0719) centre (-13, 35.0012) ccw construction
  arc A26 (-18.4117, 27.0719) -> (-17.2877, 27.9529) centre (-21.5266, 32.2036) ccw construction
  arc A27 (-17.2877, 27.9529) -> (-16.9129, 27.7382) centre (-13, 35.0012) ccw construction
  arc A28 (-16.9129, 27.7382) -> (-17.1047, 26.323) centre (-11.1024, 26.2303) ccw construction
  arc A29 (-17.1047, 26.323) -> (-16.6449, 26.12) centre (-13, 35.0012) ccw construction
  arc A30 (-16.6449, 26.12) -> (-15.7286, 27.2155) centre (-20.7586, 30.492) ccw construction
  arc A31 (-15.7286, 27.2155) -> (-15.3174, 27.0834) centre (-13, 35.0012) ccw construction
  arc A32 (-15.3174, 27.0834) -> (-15.2107, 25.6592) centre (-9.3203, 26.8165) ccw construction
  arc A33 (-15.2107, 25.6592) -> (-14.7187, 25.5563) centre (-13, 35.0012) ccw construction
  arc A34 (-14.7187, 25.5563) -> (-14.0502, 26.8183) centre (-19.6515, 28.9774) ccw construction
  arc A35 (-14.0502, 26.8183) -> (-13.6205, 26.7746) centre (-13, 35.0012) ccw construction
  arc A36 (-13.6205, 26.7746) -> (-13.2201, 25.4037) centre (-7.699, 27.7605) ccw construction
  arc A37 (-13.2201, 25.4037) -> (-12.7175, 25.4054) centre (-13, 35.0012) ccw construction
  arc A38 (-12.7175, 25.4054) -> (-12.3259, 26.7788) centre (-18.2538, 27.7261) ccw construction
  arc A39 (-12.3259, 26.7788) -> (-11.8965, 26.8253) centre (-13, 35.0012) ccw construction
  arc A40 (-11.8965, 26.8253) -> (-11.2198, 25.5677) centre (-6.3094, 29.0208) ccw construction
  arc A41 (-11.2198, 25.5677) -> (-10.7286, 25.6738) centre (-13, 35.0012) ccw construction
  arc A42 (-10.7286, 25.6738) -> (-10.6311, 27.0986) centre (-16.6264, 26.7928) ccw construction
  arc A43 (-10.6311, 27.0986) -> (-10.2208, 27.2334) centre (-13, 35.0012) ccw construction
  arc A44 (-10.2208, 27.2334) -> (-9.2974, 26.144) centre (-5.2122, 30.5426) ccw construction
  arc A45 (-9.2974, 26.144) -> (-8.8389, 26.3499) centre (-13, 35.0012) ccw construction
  arc A46 (-8.8389, 26.3499) -> (-9.0399, 27.7638) centre (-14.8405, 26.2182) ccw construction
  arc A47 (-9.0399, 27.7638) -> (-8.6665, 27.981) centre (-13, 35.0012) ccw construction
  arc A48 (-8.6665, 27.981) -> (-7.5368, 27.1073) centre (-4.4554, 32.2592) ccw construction
  arc A49 (-7.5368, 27.1073) -> (-7.1311, 27.4041) centre (-13, 35.0012) ccw construction
  arc A50 (-7.1311, 27.4041) -> (-7.6217, 28.7453) centre (-12.9742, 26.0274) ccw construction
  arc A51 (-7.6217, 28.7453) -> (-7.3016, 29.0354) centre (-13, 35.0012) ccw construction
  arc A52 (-7.3016, 29.0354) -> (-6.0149, 28.4157) centre (-4.072, 34.0956) ccw construction
  arc A53 (-6.0149, 28.4157) -> (-5.6799, 28.7903) centre (-13, 35.0012) ccw construction
  arc A54 (-5.6799, 28.7903) -> (-6.4385, 30.0002) centre (-11.109, 26.2289) ccw construction
  arc A55 (-6.4385, 30.0002) -> (-6.1858, 30.3505) centre (-13, 35.0012) ccw construction
  arc A56 (-6.1858, 30.3505) -> (-4.7984, 30.0119) centre (-4.0788, 35.9716) ccw construction
  arc A57 (-4.7984, 30.0119) -> (-4.5485, 30.448) centre (-13, 35.0012) ccw construction
  arc A58 (-4.5485, 30.448) -> (-5.5422, 31.4737) centre (-9.3265, 26.8137) ccw construction
  arc A59 (-5.5422, 31.4737) -> (-5.3678, 31.8689) centre (-13, 35.0012) ccw construction
  arc A60 (-5.3678, 31.8689) -> (-3.9403, 31.8261) centre (-4.4755, 37.8053) ccw construction
  arc A61 (-3.9403, 31.8261) -> (-3.7865, 32.3046) centre (-13, 35.0012) ccw construction
  arc A62 (-3.7865, 32.3046) -> (-4.9717, 33.1014) centre (-7.7045, 27.7564) ccw construction
  arc A63 (-4.9717, 33.1014) -> (-4.8833, 33.5242) centre (-13, 35.0012) ccw construction
  arc A64 (-4.8833, 33.5242) -> (-3.4781, 33.7791) centre (-5.2448, 39.5163) ccw construction
  arc A65 (-3.4781, 33.7791) -> (-3.4272, 34.2791) centre (-13, 35.0012) ccw construction
  arc A66 (-3.4272, 34.2791) -> (-4.7522, 34.8121) centre (-6.3139, 29.0157) ccw construction
  arc A67 (-4.7522, 34.8121) -> (-4.7536, 35.244) centre (-13, 35.0012) ccw construction
  arc A68 (-4.7536, 35.244) -> (-3.4321, 35.7855) centre (-6.353, 41.03) ccw construction
  arc A69 (-3.4321, 35.7855) -> (-3.4863, 36.2852) centre (-13, 35.0012) ccw construction
  arc A70 (-3.4863, 36.2852) -> (-4.8931, 36.531) centre (-5.2156, 30.5367) ccw construction
  arc A71 (-4.8931, 36.531) -> (-4.9843, 36.9532) centre (-13, 35.0012) ccw construction
  arc A72 (-4.9843, 36.9532) -> (-3.8043, 37.7577) centre (-7.7517, 42.2803) ccw construction
  arc A73 (-3.8043, 37.7577) -> (-3.9611, 38.2352) centre (-13, 35.0012) ccw construction
  arc A74 (-3.9611, 38.2352) -> (-5.3883, 38.1831) centre (-4.4575, 32.2527) ccw construction
  arc A75 (-5.3883, 38.1831) -> (-5.5653, 38.5771) centre (-13, 35.0012) ccw construction
  arc A76 (-5.5653, 38.5771) -> (-4.5783, 39.6094) centre (-9.3798, 43.2124) ccw construction
  arc A77 (-4.5783, 39.6094) -> (-4.831, 40.0438) centre (-13, 35.0012) ccw construction
  arc A78 (-4.831, 40.0438) -> (-6.2162, 39.6962) centre (-4.0727, 34.0888) ccw construction
  arc A79 (-6.2162, 39.6962) -> (-6.4712, 40.0448) centre (-13, 35.0012) ccw construction
  arc A80 (-6.4712, 40.0448) -> (-5.7204, 41.2596) centre (-11.1662, 43.7856) ccw construction
  arc A81 (-5.7204, 41.2596) -> (-6.0579, 41.632) centre (-13, 35.0012) ccw construction
  arc A82 (-6.0579, 41.632) -> (-7.3406, 41.004) centre (-4.0781, 35.9649) ccw construction
  arc A83 (-7.3406, 41.004) -> (-7.6625, 41.292) centre (-13, 35.0012) ccw construction
  arc A84 (-7.6625, 41.292) -> (-7.1807, 42.6364) centre (-13.0326, 43.9749) ccw construction
  arc A85 (-7.1807, 42.6364) -> (-7.5883, 42.9305) centre (-13, 35.0012) ccw construction
  arc A86 (-7.5883, 42.9305) -> (-8.7123, 42.0495) centre (-4.4734, 37.7988) ccw construction
  arc A87 (-8.7123, 42.0495) -> (-9.0871, 42.2642) centre (-13, 35.0012) ccw construction
  arc A88 (-9.0871, 42.2642) -> (-8.8953, 43.6794) centre (-14.8976, 43.7721) ccw construction
  arc A89 (-8.8953, 43.6794) -> (-9.3551, 43.8824) centre (-13, 35.0012) ccw construction
  arc A90 (-9.3551, 43.8824) -> (-10.2714, 42.7869) centre (-5.2414, 39.5104) ccw construction
  arc A91 (-10.2714, 42.7869) -> (-10.6826, 42.919) centre (-13, 35.0012) ccw construction
  arc A92 (-10.6826, 42.919) -> (-10.7893, 44.3432) centre (-16.6797, 43.1859) ccw construction
  arc A93 (-10.7893, 44.3432) -> (-11.2813, 44.4461) centre (-13, 35.0012) ccw construction
  arc A94 (-11.2813, 44.4461) -> (-11.9498, 43.1841) centre (-6.3485, 41.025) ccw construction
  arc A95 (-11.9498, 43.1841) -> (-12.3795, 43.2278) centre (-13, 35.0012) ccw construction
  arc A96 (-12.3795, 43.2278) -> (-12.7799, 44.5987) centre (-18.301, 42.2419) ccw construction
  arc A97 (-12.7799, 44.5987) -> (-13.2825, 44.597) centre (-13, 35.0012) ccw construction
  arc A98 (-13.2825, 44.597) -> (-13.6741, 43.2236) centre (-7.7462, 42.2763) ccw construction
  arc A99 (-13.6741, 43.2236) -> (-14.1035, 43.1771) centre (-13, 35.0012) ccw construction
  arc A100 (-14.1035, 43.1771) -> (-14.7802, 44.4347) centre (-19.6906, 40.9816) ccw construction
  arc A101 (-14.7802, 44.4347) -> (-15.2714, 44.3286) centre (-13, 35.0012) ccw construction
  arc A102 (-15.2714, 44.3286) -> (-15.3689, 42.9038) centre (-9.3736, 43.2096) ccw construction
  arc A103 (-15.3689, 42.9038) -> (-15.7792, 42.769) centre (-13, 35.0012) ccw construction
  arc A104 (-15.7792, 42.769) -> (-16.7026, 43.8584) centre (-20.7878, 39.4598) ccw construction
  arc A105 (-16.7026, 43.8584) -> (-17.1611, 43.6525) centre (-13, 35.0012) ccw construction
  arc A106 (-17.1611, 43.6525) -> (-16.9601, 42.2386) centre (-11.1595, 43.7842) ccw construction
  arc A107 (-16.9601, 42.2386) -> (-17.3335, 42.0214) centre (-13, 35.0012) ccw construction
  arc A108 (-17.3335, 42.0214) -> (-18.4632, 42.8951) centre (-21.5446, 37.7432) ccw construction
  arc A109 (-18.4632, 42.8951) -> (-18.8689, 42.5983) centre (-13, 35.0012) ccw construction
  arc A110 (-18.8689, 42.5983) -> (-18.3783, 41.2571) centre (-13.0258, 43.975) ccw construction
  arc A111 (-18.3783, 41.2571) -> (-18.6984, 40.967) centre (-13, 35.0012) ccw construction
  arc A112 (-18.6984, 40.967) -> (-19.9851, 41.5867) centre (-21.928, 35.9068) ccw construction
  arc A113 (-19.9851, 41.5867) -> (-20.3201, 41.2121) centre (-13, 35.0012) ccw construction
  arc A114 (-20.3201, 41.2121) -> (-19.5615, 40.0022) centre (-14.891, 43.7735) ccw construction
  arc A115 (-19.5615, 40.0022) -> (-19.8142, 39.6519) centre (-13, 35.0012) ccw construction
  arc A116 (-19.8142, 39.6519) -> (-21.2016, 39.9905) centre (-21.9212, 34.0308) ccw construction
  arc A117 (-21.2016, 39.9905) -> (-21.4515, 39.5544) centre (-13, 35.0012) ccw construction
  arc A118 (-21.4515, 39.5544) -> (-20.4578, 38.5287) centre (-16.6735, 43.1886) ccw construction
  arc A119 (-20.4578, 38.5287) -> (-20.6322, 38.1335) centre (-13, 35.0012) ccw construction
  line L0 (-6, 69.2958) -> (-9.2085, 69.2958) projected
  line L1 (-9.2085, 69.2958) -> (-9.2085, 68.7958) projected
  arc A120 (-4, 65.2958) -> (-9.2085, 68.7958) centre (-14.5, 55.2958) ccw projected
  line L2 (-4, 65.2958) -> (0, 65.2958) projected
  line L3 (0, 65.2958) -> (0, 81.4) projected
  line L4 (0, 81.4) -> (-3, 81.4) projected
  line L5 (-3, 81.4) -> (-3, 90.5) projected
  line L6 (-3, 90.5) -> (-5.4, 90.5) projected
  line L7 (-5.4, 90.5) -> (-8.7042, 87.1958) projected
  line L8 (-8.7042, 87.1958) -> (-8.7042, 86.6958) projected
  line L9 (-8.7042, 86.6958) -> (-6, 86.6958) projected
  line L10 (-6, 86.6958) -> (-6, 69.2958) projected
  circle A121 centre (-13, 35.0012) radius 9.6
  line L11 (-23.8, 30.4052) -> (-23.8, 69.2958)
  line L12 (-23.8, 69.2958) -> (-9.2085, 69.2958)
  line L13 (-4, 65.2958) -> (-23.8, 65.2958) projected
  line L14 (-4, 65.2958) -> (-23.8, 65.2958)
  circle A122 centre (-14.5, 55.2958) radius 14.5 projected
  point P0 (0, 0)
  point P1 (-25.5572, 65.2958)
  dimension "d34" = 5.2
  dimension "d36" = 1.2
  constraints: 6 end point, 2 perpendicular, 1 coincident, 1 vertical, 3 other
  measures "d34" distance edge to line of A122 L11
extrude "Extrusion4" add sketch "Sketch3" along normal blind 16.5 contours L10 L9 L8 L7 L6 L5 L4 L3 L2 A120 L1 L0 | L1 A122 L12 | A120 L13 L11 A122 L12 | A122 L11 L12
sketch "Sketch4" plane through (0, 0, -35.5) normal (0, 0, -1) x (-1, 0, 0)
  line L0 (26.0532, 64.5637) -> (22.0556, 64.7033)
  line L1 (5.4157, 65.2843) -> (22.0556, 64.7033)
  line L2 (5.4157, 65.2843) -> (1.4182, 65.4239)
  line L3 (23.8, 65.2958) -> (23.8, 69.2958)
  line L4 (23.8, 69.2958) -> (6, 69.2958)
  line L5 (6, 69.2958) -> (6, 86.6958)
  line L6 (6, 86.6958) -> (8.7042, 86.6958)
  line L7 (8.7042, 86.6958) -> (8.7042, 87.1958)
  line L8 (8.7042, 87.1958) -> (5.4, 90.5)
  line L9 (5.4, 90.5) -> (3, 90.5)
  line L10 (3, 90.5) -> (3, 81.4)
  line L11 (3, 81.4) -> (0, 81.4)
  line L12 (0, 81.4) -> (0, 65.2958)
  line L13 (0, 65.2958) -> (23.8, 65.2958)
  line L14 (1.4182, 65.4239) -> (0, 65.4735)
  line L15 (27, 52.5631) -> (27, 86.2958)
  line L16 (27, 86.2958) -> (8.7042, 87.1958)
  line L17 (27, 86.2958) -> (6.5, 86.2958)
  line L18 (26.0532, 64.5637) -> (27, 64.5306)
  line L19 (23.8, 65.2958) -> (23.8, 69.2958)
  arc A0 (18.7931, 40.8751) -> (19.3741, 42.1797) centre (13.6387, 43.9522) ccw
  arc A1 (19.3741, 42.1797) -> (18.9897, 42.5035) centre (13, 35.0012) ccw
  arc A2 (18.9897, 42.5035) -> (17.8029, 41.709) centre (21.712, 37.1532) ccw
  arc A3 (17.8029, 41.709) -> (17.4452, 41.9512) centre (13, 35.0012) ccw
  arc A4 (17.4452, 41.9512) -> (17.7423, 43.3481) centre (11.7637, 43.8894) ccw
  arc A5 (17.7423, 43.3481) -> (17.299, 43.5848) centre (13, 35.0012) ccw
  arc A6 (17.299, 43.5848) -> (16.3033, 42.561) centre (21.0742, 38.9175) ccw
  arc A7 (16.3033, 42.561) -> (15.9031, 42.7235) centre (13, 35.0012) ccw
  arc A8 (15.9031, 42.7235) -> (15.9033, 44.1517) centre (9.9428, 43.4382) ccw
  arc A9 (15.9033, 44.1517) -> (15.4204, 44.2911) centre (13, 35.0012) ccw
  arc A10 (15.4204, 44.2911) -> (14.6593, 43.0826) centre (20.0835, 40.5106) ccw
  arc A11 (14.6593, 43.0826) -> (14.2341, 43.1584) centre (13, 35.0012) ccw
  arc A12 (14.2341, 43.1584) -> (13.9373, 44.5553) centre (8.2554, 42.6182) ccw
  arc A13 (13.9373, 44.5553) -> (13.436, 44.5913) centre (13, 35.0012) ccw
  arc A14 (13.436, 44.5913) -> (12.9429, 43.251) centre (18.7832, 41.8629) ccw
  arc A15 (12.9429, 43.251) -> (12.5112, 43.2367) centre (13, 35.0012) ccw
  arc A16 (12.5112, 43.2367) -> (11.9304, 44.5414) centre (6.7755, 41.4653) ccw
  arc A17 (11.9304, 44.5414) -> (11.4326, 44.4724) centre (13, 35.0012) ccw
  arc A18 (11.4326, 44.4724) -> (11.2289, 43.0588) centre (17.2302, 42.9154) ccw
  arc A19 (11.2289, 43.0588) -> (10.8096, 42.9551) centre (13, 35.0012) ccw
  arc A20 (10.8096, 42.9551) -> (9.9703, 44.1106) centre (5.5675, 40.0299) ccw
  arc A21 (9.9703, 44.1106) -> (9.4977, 43.9395) centre (13, 35.0012) ccw
  arc A22 (9.4977, 43.9395) -> (9.5923, 42.5145) centre (15.4923, 43.622) ccw
  arc A23 (9.5923, 42.5145) -> (9.2038, 42.3259) centre (13, 35.0012) ccw
  arc A24 (9.2038, 42.3259) -> (8.1425, 43.2816) centre (4.6844, 38.3747) ccw
  arc A25 (8.1425, 43.2816) -> (7.7158, 43.016) centre (13, 35.0012) ccw
  arc A26 (7.7158, 43.016) -> (8.1047, 41.6418) centre (13.6455, 43.9518) ccw
  arc A27 (8.1047, 41.6418) -> (7.7638, 41.3765) centre (13, 35.0012) ccw
  arc A28 (7.7638, 41.3765) -> (6.5271, 42.0907) centre (4.1648, 36.572) ccw
  arc A29 (6.5271, 42.0907) -> (6.1649, 41.7423) centre (13, 35.0012) ccw
  arc A30 (6.1649, 41.7423) -> (6.831, 40.4789) centre (11.7705, 43.8904) ccw
  arc A31 (6.831, 40.4789) -> (6.5527, 40.1486) centre (13, 35.0012) ccw
  arc A32 (6.5527, 40.1486) -> (5.1945, 40.59) centre (4.0312, 34.7008) ccw
  arc A33 (5.1945, 40.59) -> (4.9127, 40.1739) centre (13, 35.0012) ccw
  arc A34 (4.9127, 40.1739) -> (5.8269, 39.0766) centre (9.9492, 43.4405) ccw
  arc A35 (5.8269, 39.0766) -> (5.6234, 38.6956) centre (13, 35.0012) ccw
  arc A36 (5.6234, 38.6956) -> (4.2031, 38.845) centre (4.2897, 32.8426) ccw
  arc A37 (4.2031, 38.845) -> (4.014, 38.3794) centre (13, 35.0012) ccw
  arc A38 (4.014, 38.3794) -> (5.1363, 37.4962) centre (8.2612, 42.6218) ccw
  arc A39 (5.1363, 37.4962) -> (5.0165, 37.0812) centre (13, 35.0012) ccw
  arc A40 (5.0165, 37.0812) -> (3.5962, 36.9321) centre (4.9288, 31.0788) ccw
  arc A41 (3.5962, 36.9321) -> (3.508, 36.4373) centre (13, 35.0012) ccw
  arc A42 (3.508, 36.4373) -> (4.7894, 35.8067) centre (6.7804, 41.47) ccw
  arc A43 (4.7894, 35.8067) -> (4.7585, 35.3759) centre (13, 35.0012) ccw
  arc A44 (4.7585, 35.3759) -> (3.4002, 34.9347) centre (5.9207, 29.4864) ccw
  arc A45 (3.4002, 34.9347) -> (3.4169, 34.4324) centre (13, 35.0012) ccw
  arc A46 (3.4169, 34.4324) -> (4.8014, 34.082) centre (5.5713, 40.0355) ccw
  arc A47 (4.8014, 34.082) -> (4.8607, 33.6542) centre (13, 35.0012) ccw
  arc A48 (4.8607, 33.6542) -> (3.6238, 32.9403) centre (7.222, 28.1351) ccw
  arc A49 (3.6238, 32.9403) -> (3.7445, 32.4524) centre (13, 35.0012) ccw
  arc A50 (3.7445, 32.4524) -> (5.1716, 32.3975) centre (4.687, 38.381) ccw
  arc A51 (5.1716, 32.3975) -> (5.3186, 31.9914) centre (13, 35.0012) ccw
  arc A52 (5.3186, 31.9914) -> (4.2572, 31.0359) centre (8.7758, 27.0838) ccw
  arc A53 (4.2572, 31.0359) -> (4.4767, 30.5838) centre (13, 35.0012) ccw
  arc A54 (4.4767, 30.5838) -> (5.884, 30.8268) centre (4.1659, 36.5788) ccw
  arc A55 (5.884, 30.8268) -> (6.1122, 30.4601) centre (13, 35.0012) ccw
  arc A56 (6.1122, 30.4601) -> (5.2727, 29.3048) centre (10.5142, 26.3786) ccw
  arc A57 (5.2727, 29.3048) -> (5.5814, 28.9082) centre (13, 35.0012) ccw
  arc A58 (5.5814, 28.9082) -> (6.9074, 29.4385) centre (4.031, 34.7076) ccw
  arc A59 (6.9074, 29.4385) -> (7.2069, 29.1273) centre (13, 35.0012) ccw
  arc A60 (7.2069, 29.1273) -> (6.6259, 27.8227) centre (12.3613, 26.0502) ccw
  arc A61 (6.6259, 27.8227) -> (7.0103, 27.4989) centre (13, 35.0012) ccw
  arc A62 (7.0103, 27.4989) -> (8.1971, 28.2934) centre (4.288, 32.8492) ccw
  arc A63 (8.1971, 28.2934) -> (8.5548, 28.0512) centre (13, 35.0012) ccw
  arc A64 (8.5548, 28.0512) -> (8.2577, 26.6543) centre (14.2363, 26.113) ccw
  arc A65 (8.2577, 26.6543) -> (8.701, 26.4176) centre (13, 35.0012) ccw
  arc A66 (8.701, 26.4176) -> (9.6967, 27.4414) centre (4.9258, 31.0849) ccw
  arc A67 (9.6967, 27.4414) -> (10.0969, 27.2789) centre (13, 35.0012) ccw
  arc A68 (10.0969, 27.2789) -> (10.0967, 25.8507) centre (16.0572, 26.5642) ccw
  arc A69 (10.0967, 25.8507) -> (10.5796, 25.7113) centre (13, 35.0012) ccw
  arc A70 (10.5796, 25.7113) -> (11.3407, 26.9198) centre (5.9165, 29.4918) ccw
  arc A71 (11.3407, 26.9198) -> (11.7659, 26.844) centre (13, 35.0012) ccw
  arc A72 (11.7659, 26.844) -> (12.0627, 25.4471) centre (17.7446, 27.3842) ccw
  arc A73 (12.0627, 25.4471) -> (12.564, 25.4111) centre (13, 35.0012) ccw
  arc A74 (12.564, 25.4111) -> (13.0571, 26.7514) centre (7.2168, 28.1395) ccw
  arc A75 (13.0571, 26.7514) -> (13.4888, 26.7657) centre (13, 35.0012) ccw
  arc A76 (13.4888, 26.7657) -> (14.0696, 25.461) centre (19.2245, 28.5371) ccw
  arc A77 (14.0696, 25.461) -> (14.5674, 25.53) centre (13, 35.0012) ccw
  arc A78 (14.5674, 25.53) -> (14.7711, 26.9436) centre (8.7698, 27.087) ccw
  arc A79 (14.7711, 26.9436) -> (15.1904, 27.0473) centre (13, 35.0012) ccw
  arc A80 (15.1904, 27.0473) -> (16.0297, 25.8918) centre (20.4325, 29.9725) ccw
  arc A81 (16.0297, 25.8918) -> (16.5023, 26.0629) centre (13, 35.0012) ccw
  arc A82 (16.5023, 26.0629) -> (16.4077, 27.4879) centre (10.5077, 26.3804) ccw
  arc A83 (16.4077, 27.4879) -> (16.7962, 27.6765) centre (13, 35.0012) ccw
  arc A84 (16.7962, 27.6765) -> (17.8575, 26.7208) centre (21.3156, 31.6277) ccw
  arc A85 (17.8575, 26.7208) -> (18.2842, 26.9864) centre (13, 35.0012) ccw
  arc A86 (18.2842, 26.9864) -> (17.8953, 28.3605) centre (12.3545, 26.0506) ccw
  arc A87 (17.8953, 28.3605) -> (18.2362, 28.6259) centre (13, 35.0012) ccw
  arc A88 (18.2362, 28.6259) -> (19.4729, 27.9117) centre (21.8352, 33.4304) ccw
  arc A89 (19.4729, 27.9117) -> (19.8351, 28.2601) centre (13, 35.0012) ccw
  arc A90 (19.8351, 28.2601) -> (19.169, 29.5235) centre (14.2295, 26.112) ccw
  arc A91 (19.169, 29.5235) -> (19.4473, 29.8538) centre (13, 35.0012) ccw
  arc A92 (19.4473, 29.8538) -> (20.8055, 29.4124) centre (21.9688, 35.3016) ccw
  arc A93 (20.8055, 29.4124) -> (21.0873, 29.8285) centre (13, 35.0012) ccw
  arc A94 (21.0873, 29.8285) -> (20.1731, 30.9258) centre (16.0508, 26.5619) ccw
  arc A95 (20.1731, 30.9258) -> (20.3766, 31.3068) centre (13, 35.0012) ccw
  arc A96 (20.3766, 31.3068) -> (21.7969, 31.1574) centre (21.7103, 37.1598) ccw
  arc A97 (21.7969, 31.1574) -> (21.986, 31.623) centre (13, 35.0012) ccw
  arc A98 (21.986, 31.623) -> (20.8637, 32.5062) centre (17.7388, 27.3806) ccw
  arc A99 (20.8637, 32.5062) -> (20.9835, 32.9212) centre (13, 35.0012) ccw
  arc A100 (20.9835, 32.9212) -> (22.4038, 33.0703) centre (21.0712, 38.9236) ccw
  arc A101 (22.4038, 33.0703) -> (22.492, 33.5651) centre (13, 35.0012) ccw
  arc A102 (22.492, 33.5651) -> (21.2106, 34.1957) centre (19.2196, 28.5324) ccw
  arc A103 (21.2106, 34.1957) -> (21.2415, 34.6265) centre (13, 35.0012) ccw
  arc A104 (21.2415, 34.6265) -> (22.5998, 35.0677) centre (20.0793, 40.516) ccw
  arc A105 (22.5998, 35.0677) -> (22.5831, 35.57) centre (13, 35.0012) ccw
  arc A106 (22.5831, 35.57) -> (21.1986, 35.9204) centre (20.4287, 29.9669) ccw
  arc A107 (21.1986, 35.9204) -> (21.1393, 36.3482) centre (13, 35.0012) ccw
  arc A108 (21.1393, 36.3482) -> (22.3762, 37.0621) centre (18.778, 41.8673) ccw
  arc A109 (22.3762, 37.0621) -> (22.2555, 37.55) centre (13, 35.0012) ccw
  arc A110 (22.2555, 37.55) -> (20.8284, 37.6049) centre (21.313, 31.6214) ccw
  arc A111 (20.8284, 37.6049) -> (20.6814, 38.011) centre (13, 35.0012) ccw
  arc A112 (20.6814, 38.011) -> (21.7428, 38.9665) centre (17.2242, 42.9186) ccw
  arc A113 (21.7428, 38.9665) -> (21.5233, 39.4186) centre (13, 35.0012) ccw
  arc A114 (21.5233, 39.4186) -> (20.116, 39.1756) centre (21.8341, 33.4236) ccw
  arc A115 (20.116, 39.1756) -> (19.8878, 39.5423) centre (13, 35.0012) ccw
  arc A116 (19.8878, 39.5423) -> (20.7273, 40.6976) centre (15.4858, 43.6238) ccw
  arc A117 (20.7273, 40.6976) -> (20.4186, 41.0942) centre (13, 35.0012) ccw
  arc A118 (20.4186, 41.0942) -> (19.0926, 40.5639) centre (21.969, 35.2948) ccw
  arc A119 (19.0926, 40.5639) -> (18.7931, 40.8751) centre (13, 35.0012) ccw
  circle A120 centre (14.5, 55.2958) radius 14.5
  circle A121 centre (14.5, 55.2958) radius 13.85
  line L20 (23.8, 65.2958) -> (27, 65.2958)
  line L21 (23.8, 69.2958) -> (27, 69.2958)
  point P0 (0, 0)
  point P1 (5.0862, 65.2958)
  point P2 (4, 65.2958)
  point P3 (4.0351, 65.3325)
  point P4 (4.9176, 65.2958)
  point P5 (4.9235, 65.3015)
extrude "Extrusion7" add sketch "Sketch4" along normal blind 14.5 contours L20 A121 L3 A120 | A120 L3 L21 L15 L20 | L20 L3 A121 | A120 L4 L3 | L3 A121 L2 A120 L4 | L21 L4 A120 L5 L6 L7 L16 L15 | L3 L13 L2 A121 | L4 A120 | A120 L2 L14 L12 L11 L10 L9 L8 L7 L6 L5 L4
ref_plane "Work Plane4" through (-23.1368, 52.6716, -30.5) normal (0, 0, 1) x (0.9993908, 0.0348995, 0)
extrude "Extrusion8" add sketch "Sketch4" against normal up to surface (5 mm away) contours L20 A121 L3 A120 | A120 L3 L21 L15 L20 | L20 L3 A121
ref_plane "Work Plane5" through (-23.1368, 52.6716, -30.5) normal (0, 0, 1) x (0.9993908, 0.0348995, 0)
extrude "Extrusion9" cut sketch "Sketch4" against normal up to surface (5 mm away) contours L13 A120 L2 | A120 L13 L12 L14 L2